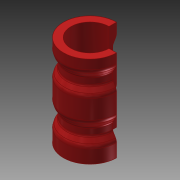
# Autodesk Inventor part: Foam Weight Shifter Pad 2
Saved by Autodesk Inventor 2014 SP1 (Build 180222100, 222)
## iProperties
Created: 2013-12-18
Part Number: Foam Weight Shifter Pad 2
Material: Generic
Document SubType Name: Modeling
Designer: Moses
Mass: 90.7185 g
Surface Area: 794.271 cm^2
Volume: 405.265 cm^3
Density: 0.22385 g/cm^3
Appearance: Light Red
Author: Moses
Autodesk Inventor part; units mm, degrees
ref_plane "YZ Plane" through (0, 0, 0) normal (1, 0, 0) x (0, 1, 0)
ref_plane "XZ Plane" through (0, 0, 0) normal (0, 1, 0) x (-1, 0, 0)
ref_plane "XY Plane" through (0, 0, 0) normal (0, 0, 1) x (1, 0, 0)
sketch "Sketch1" plane through (0, 0, 0) normal (0, 0, 1) x (1, 0, 0)
  line L0 (0, 0) -> (31.75, 0) construction
  line L1 (31.75, 0) -> (44.45, 0)
  line L2 (44.45, 0) -> (44.45, -19.05)
  line L3 (44.45, -19.05) -> (38.1, -30.0485)
  line L4 (38.1, -30.0485) -> (38.1, -42.7485)
  line L5 (38.1, -42.7485) -> (44.45, -53.747)
  line L6 (44.45, -53.747) -> (44.45, -92.303)
  line L7 (44.45, -92.303) -> (38.1, -103.3015)
  line L8 (38.1, -103.3015) -> (38.1, -116.0015)
  line L9 (38.1, -116.0015) -> (44.45, -127)
  line L10 (44.45, -127) -> (44.45, -152.4)
  line L11 (44.45, -152.4) -> (31.75, -152.4)
  line L12 (31.75, -152.4) -> (31.75, 0)
  line L13 (0, 0) -> (0, -152.4)
  dimension "d0" = 31.75
  dimension "d1" = 12.7
  dimension "d2" = 6.35
  dimension "d3" = 150
  dimension "d4" = 19.05
  dimension "d5" = 152.4
  dimension "d6" = 150
  dimension "d7" = 12.7
  dimension "d8" = 25.4
  dimension "d9" = 152.4
  constraints: 28 end point, 7 vertical, 4 equal length, 3 horizontal, 2 parallel
  measures "d0" distance of L0.start L0.end
  measures "d1" distance of L0.end L1.end
  measures "d2" horizontal distance of L2.end L3.end
  measures "d3" angle of L2 L3
  measures "d4" distance of L1.end L2.end
  measures "d5" distance of L11.end L0.end
  measures "d6" angle of L5 L6
  measures "d7" distance of L3.end L4.end
  measures "d8" distance from line of L11 L9.end
  measures "d9" distance of L0.start L13.end
revolve "Revolution1" add sketch "Sketch1" angle 270 about axis through (0, 0, 0) along (0, -1, 0)
fillet "Fillet1" radius 12.7 4 edges at (-31.4309, -19.05, 31.4309) (-31.4309, -53.747, 31.4309) (-31.4309, -92.303, 31.4309) (-31.4309, -127, 31.4309)
fillet "Fillet1" radius 6.35 4 edges at (-26.9408, -42.7485, 26.9408) (-26.9408, -30.0485, 26.9408) (-26.9408, -103.3015, 26.9408) (-26.9408, -116.0015, 26.9408)
equation "\"d6\" = d3"
body "Solid1"
